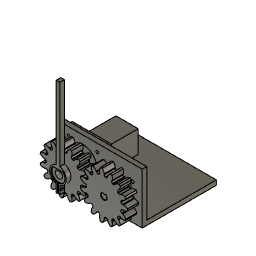
Encoder v10 (Autodesk Fusion 360 design; units mm, degrees)
description: Spur Gear; Module: 3.0; Num Teeth: 15; Pressure Angle: 20.0; Backlash: 0.00 mm
Autodesk Fusion 360 part; units mm, degrees
(part 1 of 6)
sketch "Sketch1" plane through (0, 0, 0) normal (0, 1, 0) x (1, 0, 0) in component "Motor"
  line L0 (0, 0) -> (-21.175, 0) construction
  line L1 (-21.175, 0) -> (-21.175, 21.175) construction
  line L2 (-21.175, 21.175) -> (0, 21.175) construction
  line L3 (0, 21.175) -> (0, 0) construction
  line L4 (-21.175, 21.175) -> (21.175, 21.175)
  line L5 (21.175, 21.175) -> (21.175, -21.175)
  line L6 (21.175, -21.175) -> (-21.175, -21.175)
  line L7 (-21.175, -21.175) -> (-21.175, 21.175)
  line L8 (0, 0) -> (-15.5, 0) construction
  line L9 (-15.5, 0) -> (-15.5, 15.5) construction
  line L10 (-15.5, 15.5) -> (0, 15.5) construction
  line L11 (0, 15.5) -> (0, 0) construction
  line L12 (-15.5, 15.5) -> (15.5, 15.5) construction
  line L13 (15.5, 15.5) -> (15.5, -15.5) construction
  line L14 (15.5, -15.5) -> (-15.5, -15.5) construction
  line L15 (-15.5, -15.5) -> (-15.5, 15.5) construction
  circle A0 centre (-15.5, 15.5) radius 1.5
  circle A1 centre (15.5, 15.5) radius 1.5
  circle A2 centre (-15.5, -15.5) radius 1.5
  circle A3 centre (15.5, -15.5) radius 1.5
  dimension "d68" = 21.175
  dimension "d69" = 21.175
  dimension "d70" = 42.35
  dimension "d71" = 42.35
  dimension "d72" = 15.5
  dimension "d73" = 15.5
  dimension "d74" = 31
  dimension "d75" = 31
  dimension "d76" = 3
  dimension "d77" = 3
  dimension "d78" = 3
  dimension "d79" = 3
  constraint horizontal L0
  constraint vertical L1
  constraint horizontal L2
  constraint vertical L3
  constraint coincident L0.start L3.end
  constraint horizontal L4
  constraint vertical L5
  constraint horizontal L6
  constraint vertical L7
  constraint horizontal L8
  constraint vertical L9
  constraint horizontal L10
  constraint vertical L11
  constraint horizontal L12
  constraint vertical L13
  constraint horizontal L14
  constraint vertical L15
  constraint coincident L9.end L10.start
  constraint coincident L12.end L13.start
  constraint coincident L14.end L15.start
  constraint coincident L13.end L14.start
  measures "d68" distance of L0.start L0.end
  measures "d69" distance of L0.start L2.end
  measures "d70" distance of L1.end L4.end
  measures "d71" distance of L1.end L6.end
  measures "d72" distance of L0.start L8.end
  measures "d73" distance of L0.start L10.end
  measures "d74" distance of L9.end L12.end
  measures "d75" distance of L9.end L14.end
  measures "d76" diameter of A0
  measures "d77" diameter of A1
  measures "d78" diameter of A2
  measures "d79" diameter of A3
extrude "Extrude1" add sketch "Sketch1" along normal blind 4.5 makes body 1 in component "Motor"
sketch "Sketch2" plane through (0, 4.5, 0) normal (0, 1, 0) x (-1, 0, 0) in component "Motor"
  circle A0 centre (15.5, -15.5) radius 1.5
  circle A1 centre (15.5, 15.5) radius 1.5
  circle A2 centre (-15.5, -15.5) radius 1.5
  circle A3 centre (-15.5, 15.5) radius 1.5
  line L0 (21.175, 21.175) -> (-21.175, 21.175)
  line L1 (-21.175, 21.175) -> (-21.175, -21.175)
  line L2 (-21.175, -21.175) -> (21.175, -21.175)
  line L3 (21.175, -21.175) -> (21.175, 21.175)
  line L4 (0, 0) -> (-12, 0) construction
  line L5 (-12, 0) -> (-12, -12) construction
  line L6 (-12, -12) -> (0, -12) construction
  line L7 (0, -12) -> (0, 0) construction
  line L8 (-12, -12) -> (12, -12)
  line L9 (12, -12) -> (12, 12)
  line L10 (12, 12) -> (-12, 12)
  line L11 (-12, 12) -> (-12, -12)
  dimension "d82" = 12
  dimension "d83" = 12
  dimension "d84" = 24
  dimension "d85" = 24
  constraint horizontal L4
  constraint vertical L5
  constraint horizontal L6
  constraint vertical L7
  constraint coincident L4.start L7.end
  constraint horizontal L8
  constraint vertical L9
  constraint horizontal L10
  constraint vertical L11
  measures "d82" distance of L4.start L4.end
  measures "d83" distance of L4.start L6.end
  measures "d84" distance of L5.end L8.end
  measures "d85" distance of L5.end L10.end
extrude "Extrude2" add sketch "Sketch2" along normal blind 38 contours L8 L9 L10 L11 bodies 1 in component "Motor"
sketch "Sketch3" plane through (0, 0, 0) normal (0, -1, 0) x (1, 0, 0) in component "Motor"
  circle A0 centre (-15.5, -15.5) radius 1.5
  circle A1 centre (-15.5, 15.5) radius 1.5
  circle A2 centre (15.5, -15.5) radius 1.5
  circle A3 centre (15.5, 15.5) radius 1.5
  line L0 (21.175, 21.175) -> (-21.175, 21.175)
  line L1 (-21.175, 21.175) -> (-21.175, -21.175)
  line L2 (-21.175, -21.175) -> (21.175, -21.175)
  line L3 (21.175, -21.175) -> (21.175, 21.175)
  circle A4 centre (0, 0) radius 12
  dimension "d88" = 24
  constraint coincident A4.centre origin
  measures "d88" diameter of A4
extrude "Extrude3" add sketch "Sketch3" along normal blind 2 contours A4 bodies 1 in component "Motor"
sketch "Sketch4" plane through (0, -2, 0) normal (0, -1, 0) x (1, 0, 0) in component "Motor"
  circle A0 centre (0, 0) radius 12
  circle A1 centre (0, 0) radius 4
  dimension "d91" = 8
  constraint coincident A0.centre A1.centre
  measures "d91" diameter of A1
extrude "Extrude4" add sketch "Sketch4" along normal blind 20 contours A1 bodies 1 in component "Motor"
sketch "Sketch1 (2)" plane through (0, 0, 0) normal (0, 1, 0) x (1, 0, 0) in component "encoder"
  line L0 (0, 0) -> (19, 0)
  line L1 (19, 0) -> (19, -26)
  line L2 (19, -26) -> (0, -26)
  line L3 (0, -26) -> (0, 0)
  line L4 (0, 0) -> (8, 0) construction
  line L5 (8, 0) -> (8, -12) construction
  line L6 (8, -12) -> (0, -12) construction
  line L7 (0, -12) -> (0, 0) construction
  line L8 (8, -12) -> (2.5, -12) construction
  line L9 (2.5, -12) -> (2.5, -6) construction
  line L10 (2.5, -6) -> (8, -6) construction
  line L11 (8, -6) -> (8, -12) construction
  line L12 (2.5, -6) -> (13.5, -6)
  line L13 (13.5, -6) -> (13.5, -18)
  line L14 (13.5, -18) -> (2.5, -18)
  line L15 (2.5, -18) -> (2.5, -6)
  dimension "d94" = 19
  dimension "d95" = 26
  dimension "d96" = 8
  dimension "d97" = 12
  dimension "d98" = 5.5
  dimension "d99" = 6
  dimension "d100" = 11
  dimension "d101" = 12
  constraint horizontal L0
  constraint vertical L1
  constraint horizontal L2
  constraint vertical L3
  constraint coincident L0.start L3.end
  constraint horizontal L4
  constraint vertical L5
  constraint horizontal L6
  constraint vertical L7
  constraint horizontal L8
  constraint vertical L9
  constraint horizontal L10
  constraint vertical L11
  constraint horizontal L12
  constraint vertical L13
  constraint horizontal L14
  constraint vertical L15
  measures "d94" distance of L0.start L0.end
  measures "d95" distance of L0.start L2.end
  measures "d96" distance of L0.start L4.end
  measures "d97" distance of L0.start L6.end
  measures "d98" distance of L5.end L8.end
  measures "d99" distance of L5.end L10.end
  measures "d100" distance of L9.end L12.end
  measures "d101" distance of L9.end L14.end
extrude "Extrude1'" add sketch "Sketch1 (2)" against normal blind 7 separate body contours L12 L13 L14 L15 makes body 2 in component "encoder"
extrude "Extrude2'" add sketch "Sketch1 (2)" along normal blind 1.2 separate body makes body 3 in component "encoder"
sketch "Sketch2 (2)" plane through (0, -7, 0) normal (0, -1, 0) x (1, 0, 0) in component "encoder"
  line L0 (13.5, 18) -> (2.5, 18)
  line L1 (2.5, 18) -> (2.5, 6)
  line L2 (2.5, 6) -> (13.5, 6)
  line L3 (13.5, 6) -> (13.5, 18)
  line L4 (2.5, 18) -> (13.5, 6) construction
  circle A0 centre (8, 12) radius 3
  dimension "d106" = 6
  constraint coincident L0.end L1.start
  constraint coincident L2.end L3.start
  constraint midpoint L4 A0.centre
  measures "d106" diameter of A0
extrude "Extrude3'" add sketch "Sketch2 (2)" along normal blind 20 contours A0 bodies 2 in component "encoder"
sketch "Sketch1 (3)" plane through (0, 0, 0) normal (0, 0, 1) x (1, 0, 0) in component "Spur Gear (15 teeth) (1)"
  circle A0 centre (0, 0) radius 18.8492
  circle A1 centre (0, 0) radius 4
extrude "Extrude1''" add sketch "Sketch1 (3)" along normal blind 12 separate body makes body 4 in component "Spur Gear (15 teeth) (1)"
sketch "Sketch2 (3)" plane through (0, 0, 0) normal (0, 0, 1) x (1, 0, 0) in component "Spur Gear (15 teeth) (1)"
  spline S0 degree 5 poles (20.992, -2.5232) (21.0048, -2.5247) (21.0305, -2.5274) (21.0691, -2.5303) (21.1207, -2.5321) (21.1854, -2.5313) (21.2502, -2.5284) (21.315, -2.5242) (21.38, -2.5193) (21.4449, -2.5139) (21.5099, -2.508) (21.575, -2.5014) (21.64, -2.4939) (21.7051, -2.4854) (21.7702, -2.4759) (21.8353, -2.4653) (21.9004, -2.454) (21.9656, -2.442) (22.0307, -2.4293) (22.0958, -2.4161) (22.1609, -2.4023) (22.226, -2.3879) (22.2911, -2.3729) (22.3562, -2.3572) (22.4212, -2.3409) (22.4862, -2.324) (22.5512, -2.3064) (22.6162, -2.2883) (22.6811, -2.2697) (22.746, -2.2505) (22.8109, -2.2308) (22.8757, -2.2106) (22.9405, -2.1898) (23.0053, -2.1685) (23.07, -2.1467) (23.1347, -2.1244) (23.1993, -2.1016) (23.2639, -2.0783) (23.3284, -2.0545) (23.3929, -2.0302) (23.4573, -2.0055) (23.5217, -1.9803) (23.586, -1.9546) (23.6502, -1.9284) (23.7144, -1.9018) (23.7785, -1.8747) (23.8426, -1.8472) (23.9066, -1.8192) (23.9705, -1.7908) (24.0344, -1.762) (24.0982, -1.7327) (24.1619, -1.703) (24.2255, -1.6729) (24.2891, -1.6423) (24.3526, -1.6113) (24.416, -1.5799) (24.4793, -1.5481) (24.5426, -1.5158) (24.6058, -1.4832) (24.6689, -1.4501) (24.7319, -1.4166) (24.7948, -1.3828) (24.8577, -1.3485) (24.9204, -1.3139) (24.9831, -1.2788) (25.0457, -1.2434) (25.1081, -1.2075) (25.1705, -1.1713) (25.2328, -1.1347) (25.295, -1.0977) (25.3571, -1.0603) (25.4067, -1.0301) (25.4439, -1.0073) (25.4686, -0.992) (25.481, -0.9843) knots 0 0 0 0 0 0 0.01428571 0.02857143 0.04285714 0.05714286 0.07142857 0.08571429 0.1 0.11428571 0.12857143 0.14285714 0.15714286 0.17142857 0.18571429 0.2 0.21428571 0.22857143 0.24285714 0.25714286 0.27142857 0.28571429 0.3 0.31428571 0.32857143 0.34285714 0.35714286 0.37142857 0.38571429 0.4 0.41428571 0.42857143 0.44285714 0.45714286 0.47142857 0.48571429 0.5 0.51428571 0.52857143 0.54285714 0.55714286 0.57142857 0.58571429 0.6 0.61428571 0.62857143 0.64285714 0.65714286 0.67142857 0.68571429 0.7 0.71428571 0.72857143 0.74285714 0.75714286 0.77142857 0.78571429 0.8 0.81428571 0.82857143 0.84285714 0.85714286 0.87142857 0.88571429 0.9 0.91428571 0.92857143 0.94285714 0.95714286 0.97142857 0.98571429 1 1 1 1 1 1
  spline S1 degree 5 poles (20.992, 2.5232) (21.0048, 2.5247) (21.0305, 2.5274) (21.0691, 2.5303) (21.1207, 2.5321) (21.1854, 2.5313) (21.2502, 2.5284) (21.315, 2.5242) (21.38, 2.5193) (21.4449, 2.5139) (21.5099, 2.508) (21.575, 2.5014) (21.64, 2.4939) (21.7051, 2.4854) (21.7702, 2.4759) (21.8353, 2.4653) (21.9004, 2.454) (21.9656, 2.442) (22.0307, 2.4293) (22.0958, 2.4161) (22.1609, 2.4023) (22.226, 2.3879) (22.2911, 2.3729) (22.3562, 2.3572) (22.4212, 2.3409) (22.4862, 2.324) (22.5512, 2.3064) (22.6162, 2.2883) (22.6811, 2.2697) (22.746, 2.2505) (22.8109, 2.2308) (22.8757, 2.2106) (22.9405, 2.1898) (23.0053, 2.1685) (23.07, 2.1467) (23.1347, 2.1244) (23.1993, 2.1016) (23.2639, 2.0783) (23.3284, 2.0545) (23.3929, 2.0302) (23.4573, 2.0055) (23.5217, 1.9803) (23.586, 1.9546) (23.6502, 1.9284) (23.7144, 1.9018) (23.7785, 1.8747) (23.8426, 1.8472) (23.9066, 1.8192) (23.9705, 1.7908) (24.0344, 1.762) (24.0982, 1.7327) (24.1619, 1.703) (24.2255, 1.6729) (24.2891, 1.6423) (24.3526, 1.6113) (24.416, 1.5799) (24.4793, 1.5481) (24.5426, 1.5158) (24.6058, 1.4832) (24.6689, 1.4501) (24.7319, 1.4166) (24.7948, 1.3828) (24.8577, 1.3485) (24.9204, 1.3139) (24.9831, 1.2788) (25.0457, 1.2434) (25.1081, 1.2075) (25.1705, 1.1713) (25.2328, 1.1347) (25.295, 1.0977) (25.3571, 1.0603) (25.4067, 1.0301) (25.4439, 1.0073) (25.4686, 0.992) (25.481, 0.9843) knots 0 0 0 0 0 0 0.01428571 0.02857143 0.04285714 0.05714286 0.07142857 0.08571429 0.1 0.11428571 0.12857143 0.14285714 0.15714286 0.17142857 0.18571429 0.2 0.21428571 0.22857143 0.24285714 0.25714286 0.27142857 0.28571429 0.3 0.31428571 0.32857143 0.34285714 0.35714286 0.37142857 0.38571429 0.4 0.41428571 0.42857143 0.44285714 0.45714286 0.47142857 0.48571429 0.5 0.51428571 0.52857143 0.54285714 0.55714286 0.57142857 0.58571429 0.6 0.61428571 0.62857143 0.64285714 0.65714286 0.67142857 0.68571429 0.7 0.71428571 0.72857143 0.74285714 0.75714286 0.77142857 0.78571429 0.8 0.81428571 0.82857143 0.84285714 0.85714286 0.87142857 0.88571429 0.9 0.91428571 0.92857143 0.94285714 0.95714286 0.97142857 0.98571429 1 1 1 1 1 1
  arc A0 (25.481, -0.9843) -> (25.481, 0.9843) centre (0, 0) ccw
  line L0 (18.7046, -2.2494) -> (20.992, -2.5232)
  line L1 (18.7046, 2.2494) -> (20.992, 2.5232)
  line L2 (18.7046, -2.2494) -> (18.7046, 2.2494)
  point P0 (21.3052, -2.5247)
  point P1 (21.6219, -2.4959)
  point P2 (21.9407, -2.4465)
  point P3 (22.2611, -2.3798)
  point P4 (22.5825, -2.2976)
  point P5 (22.9048, -2.2012)
  point P6 (23.2276, -2.0913)
  point P7 (23.5506, -1.9686)
  point P8 (23.8736, -1.8336)
  point P9 (24.1965, -1.6866)
  point P10 (24.5188, -1.5279)
  point P11 (24.8405, -1.3578)
  point P12 (25.1613, -1.1766)
  point P13 (21.3052, 2.5247)
  point P14 (21.6219, 2.4959)
  point P15 (21.9407, 2.4465)
  point P16 (22.2611, 2.3798)
  point P17 (22.5825, 2.2976)
  point P18 (22.9048, 2.2012)
  point P19 (23.2276, 2.0913)
  point P20 (23.5506, 1.9686)
  point P21 (23.8736, 1.8336)
  point P22 (24.1965, 1.6866)
  point P23 (24.5188, 1.5279)
  point P24 (24.8405, 1.3578)
  point P25 (25.1613, 1.1766)
extrude "Extrude2''" add sketch "Sketch2 (3)" along normal blind 12 bodies 4 in component "Spur Gear (15 teeth) (1)"
fillet "Fillet1" radius 1.5 2 edges at (18.7144, -2.2506, 6) (18.7144, 2.2506, 6) on bodies 4 in component "Spur Gear (15 teeth) (1)"
pattern_circular "C-Pattern1" count 15 over 360 about axis through (0, 0, 0) along (0, 0, 1) of "Extrude2''", "Fillet1" in component "Spur Gear (15 teeth) (1)"
sketch "Sketch3 (2)" plane through (0, 0, 0) normal (0, 0, 1) x (1, 0, 0) in component "Spur Gear (15 teeth) (1)"
  circle A0 centre (0, 0) radius 22.5 construction
sketch "Sketch1 (4)" plane through (0, 0, 0) normal (0, 0, 1) x (1, 0, 0) in component "Spur Gear (15 teeth)"
  circle A0 centre (0, 0) radius 18.8492
  circle A1 centre (0, 0) radius 3.5
  dimension "d237" = 7
  measures "d237" diameter of A1
extrude "Extrude1'''" add sketch "Sketch1 (4)" along normal blind 12 separate body makes body 5 in component "Spur Gear (15 teeth)"
sketch "Sketch2 (4)" plane through (0, 0, 0) normal (0, 0, 1) x (1, 0, 0) in component "Spur Gear (15 teeth)"
  spline S0 degree 5 poles (20.992, -2.5232) (21.0048, -2.5247) (21.0305, -2.5274) (21.0691, -2.5303) (21.1207, -2.5321) (21.1854, -2.5313) (21.2502, -2.5284) (21.315, -2.5242) (21.38, -2.5193) (21.4449, -2.5139) (21.5099, -2.508) (21.575, -2.5014) (21.64, -2.4939) (21.7051, -2.4854) (21.7702, -2.4759) (21.8353, -2.4653) (21.9004, -2.454) (21.9656, -2.442) (22.0307, -2.4293) (22.0958, -2.4161) (22.1609, -2.4023) (22.226, -2.3879) (22.2911, -2.3729) (22.3562, -2.3572) (22.4212, -2.3409) (22.4862, -2.324) (22.5512, -2.3064) (22.6162, -2.2883) (22.6811, -2.2697) (22.746, -2.2505) (22.8109, -2.2308) (22.8757, -2.2106) (22.9405, -2.1898) (23.0053, -2.1685) (23.07, -2.1467) (23.1347, -2.1244) (23.1993, -2.1016) (23.2639, -2.0783) (23.3284, -2.0545) (23.3929, -2.0302) (23.4573, -2.0055) (23.5217, -1.9803) (23.586, -1.9546) (23.6502, -1.9284) (23.7144, -1.9018) (23.7785, -1.8747) (23.8426, -1.8472) (23.9066, -1.8192) (23.9705, -1.7908) (24.0344, -1.762) (24.0982, -1.7327) (24.1619, -1.703) (24.2255, -1.6729) (24.2891, -1.6423) (24.3526, -1.6113) (24.416, -1.5799) (24.4793, -1.5481) (24.5426, -1.5158) (24.6058, -1.4832) (24.6689, -1.4501) (24.7319, -1.4166) (24.7948, -1.3828) (24.8577, -1.3485) (24.9204, -1.3139) (24.9831, -1.2788) (25.0457, -1.2434) (25.1081, -1.2075) (25.1705, -1.1713) (25.2328, -1.1347) (25.295, -1.0977) (25.3571, -1.0603) (25.4067, -1.0301) (25.4439, -1.0073) (25.4686, -0.992) (25.481, -0.9843) knots 0 0 0 0 0 0 0.01428571 0.02857143 0.04285714 0.05714286 0.07142857 0.08571429 0.1 0.11428571 0.12857143 0.14285714 0.15714286 0.17142857 0.18571429 0.2 0.21428571 0.22857143 0.24285714 0.25714286 0.27142857 0.28571429 0.3 0.31428571 0.32857143 0.34285714 0.35714286 0.37142857 0.38571429 0.4 0.41428571 0.42857143 0.44285714 0.45714286 0.47142857 0.48571429 0.5 0.51428571 0.52857143 0.54285714 0.55714286 0.57142857 0.58571429 0.6 0.61428571 0.62857143 0.64285714 0.65714286 0.67142857 0.68571429 0.7 0.71428571 0.72857143 0.74285714 0.75714286 0.77142857 0.78571429 0.8 0.81428571 0.82857143 0.84285714 0.85714286 0.87142857 0.88571429 0.9 0.91428571 0.92857143 0.94285714 0.95714286 0.97142857 0.98571429 1 1 1 1 1 1
  spline S1 degree 5 poles (20.992, 2.5232) (21.0048, 2.5247) (21.0305, 2.5274) (21.0691, 2.5303) (21.1207, 2.5321) (21.1854, 2.5313) (21.2502, 2.5284) (21.315, 2.5242) (21.38, 2.5193) (21.4449, 2.5139) (21.5099, 2.508) (21.575, 2.5014) (21.64, 2.4939) (21.7051, 2.4854) (21.7702, 2.4759) (21.8353, 2.4653) (21.9004, 2.454) (21.9656, 2.442) (22.0307, 2.4293) (22.0958, 2.4161) (22.1609, 2.4023) (22.226, 2.3879) (22.2911, 2.3729) (22.3562, 2.3572) (22.4212, 2.3409) (22.4862, 2.324) (22.5512, 2.3064) (22.6162, 2.2883) (22.6811, 2.2697) (22.746, 2.2505) (22.8109, 2.2308) (22.8757, 2.2106) (22.9405, 2.1898) (23.0053, 2.1685) (23.07, 2.1467) (23.1347, 2.1244) (23.1993, 2.1016) (23.2639, 2.0783) (23.3284, 2.0545) (23.3929, 2.0302) (23.4573, 2.0055) (23.5217, 1.9803) (23.586, 1.9546) (23.6502, 1.9284) (23.7144, 1.9018) (23.7785, 1.8747) (23.8426, 1.8472) (23.9066, 1.8192) (23.9705, 1.7908) (24.0344, 1.762) (24.0982, 1.7327) (24.1619, 1.703) (24.2255, 1.6729) (24.2891, 1.6423) (24.3526, 1.6113) (24.416, 1.5799) (24.4793, 1.5481) (24.5426, 1.5158) (24.6058, 1.4832) (24.6689, 1.4501) (24.7319, 1.4166) (24.7948, 1.3828) (24.8577, 1.3485) (24.9204, 1.3139) (24.9831, 1.2788) (25.0457, 1.2434) (25.1081, 1.2075) (25.1705, 1.1713) (25.2328, 1.1347) (25.295, 1.0977) (25.3571, 1.0603) (25.4067, 1.0301) (25.4439, 1.0073) (25.4686, 0.992) (25.481, 0.9843) knots 0 0 0 0 0 0 0.01428571 0.02857143 0.04285714 0.05714286 0.07142857 0.08571429 0.1 0.11428571 0.12857143 0.14285714 0.15714286 0.17142857 0.18571429 0.2 0.21428571 0.22857143 0.24285714 0.25714286 0.27142857 0.28571429 0.3 0.31428571 0.32857143 0.34285714 0.35714286 0.37142857 0.38571429 0.4 0.41428571 0.42857143 0.44285714 0.45714286 0.47142857 0.48571429 0.5 0.51428571 0.52857143 0.54285714 0.55714286 0.57142857 0.58571429 0.6 0.61428571 0.62857143 0.64285714 0.65714286 0.67142857 0.68571429 0.7 0.71428571 0.72857143 0.74285714 0.75714286 0.77142857 0.78571429 0.8 0.81428571 0.82857143 0.84285714 0.85714286 0.87142857 0.88571429 0.9 0.91428571 0.92857143 0.94285714 0.95714286 0.97142857 0.98571429 1 1 1 1 1 1
  arc A0 (25.481, -0.9843) -> (25.481, 0.9843) centre (0, 0) ccw
  line L0 (18.7046, -2.2494) -> (20.992, -2.5232)
  line L1 (18.7046, 2.2494) -> (20.992, 2.5232)
  line L2 (18.7046, -2.2494) -> (18.7046, 2.2494)
  point P0 (21.3052, -2.5247)
  point P1 (21.6219, -2.4959)
  point P2 (21.9407, -2.4465)
  point P3 (22.2611, -2.3798)
  point P4 (22.5825, -2.2976)
  point P5 (22.9048, -2.2012)
  point P6 (23.2276, -2.0913)
  point P7 (23.5506, -1.9686)
  point P8 (23.8736, -1.8336)
  point P9 (24.1965, -1.6866)
  point P10 (24.5188, -1.5279)
  point P11 (24.8405, -1.3578)
  point P12 (25.1613, -1.1766)
  point P13 (21.3052, 2.5247)
  point P14 (21.6219, 2.4959)
  point P15 (21.9407, 2.4465)
  point P16 (22.2611, 2.3798)
  point P17 (22.5825, 2.2976)
  point P18 (22.9048, 2.2012)
  point P19 (23.2276, 2.0913)
  point P20 (23.5506, 1.9686)
  point P21 (23.8736, 1.8336)
  point P22 (24.1965, 1.6866)
  point P23 (24.5188, 1.5279)
  point P24 (24.8405, 1.3578)
  point P25 (25.1613, 1.1766)
extrude "Extrude2'''" add sketch "Sketch2 (4)" along normal blind 12 bodies 5 in component "Spur Gear (15 teeth)"
fillet "Fillet1'" radius 1.5 2 edges at (18.7144, -2.2506, 6) (18.7144, 2.2506, 6) on bodies 5 in component "Spur Gear (15 teeth)"
pattern_circular "C-Pattern1'" count 15 over 360 about axis through (0, 0, 0) along (0, 0, 1) of "Extrude2'''", "Fillet1'" in component "Spur Gear (15 teeth)"
sketch "Sketch3 (3)" plane through (0, 0, 0) normal (0, 0, 1) x (1, 0, 0) in component "Spur Gear (15 teeth)"
  circle A0 centre (0, 0) radius 22.5 construction
sketch "Sketch1 (5)" plane through (0, 0, 0) normal (0, -1, 0) x (1, 0, 0) in component "Body"
  circle A0 centre (0, 0) radius 12
  circle A1 centre (-15.5, -15.5) radius 1.5
  circle A2 centre (-15.5, 15.5) radius 1.5
  circle A3 centre (15.5, -15.5) radius 1.5
  circle A4 centre (15.5, 15.5) radius 1.5
  line L0 (21.175, 21.175) -> (-21.175, 21.175)
  line L1 (-21.175, 21.175) -> (-21.175, -21.175)
  line L2 (-21.175, -21.175) -> (21.175, -21.175)
  line L3 (21.175, -21.175) -> (21.175, 21.175)
  line L4 (-21.175, -21.175) -> (-26.175, -21.175) construction
  line L5 (-26.175, -21.175) -> (-26.175, -26.175) construction
  line L6 (-26.175, -26.175) -> (-21.175, -26.175) construction
  line L7 (-21.175, -26.175) -> (-21.175, -21.175) construction
  line L8 (-26.175, -26.175) -> (63.825, -26.175)
  line L9 (63.825, -26.175) -> (63.825, 23.825)
  line L10 (63.825, 23.825) -> (-26.175, 23.825)
  line L11 (-26.175, 23.825) -> (-26.175, -26.175)
  dimension "d141" = 5
  dimension "d142" = 5
  dimension "d143" = 90
  dimension "d144" = 50
  constraint horizontal L4
  constraint vertical L5
  constraint horizontal L6
  constraint vertical L7
  constraint coincident L1.end L2.start
  constraint horizontal L8
  constraint vertical L9
  constraint horizontal L10
  constraint vertical L11
  measures "d141" distance of L1.end L4.end
  measures "d142" distance of L1.end L6.end
  measures "d143" distance of L5.end L8.end
  measures "d144" distance of L5.end L10.end
extrude "Extrude1''''" add sketch "Sketch1 (5)" against normal blind 5 separate body contours A0 | L0 L1 L2 L3 | L8 L9 L10 L11 makes body 6 in component "Body"
sketch "Sketch2 (5)" plane through (0, -11, 0) normal (0, -1, 0) x (1, 0, 0) in component "Body"
  circle A0 centre (0, 0) radius 4
  circle A1 centre (0, 0) radius 15
  dimension "d147" = 30
  constraint coincident A0.centre A1.centre
  measures "d147" diameter of A1
extrude "Extrude2''''" cut sketch "Sketch2 (5)" against normal blind 16 contours A0 | A1 bodies 6 in component "Body"
sketch "Sketch3 (4)" plane through (0, 8.3, 0) normal (0, 1, 0) x (-1, 0, 0) in component "Body"
  line L0 (-39.2194, 6) -> (-50.2194, 6)
  line L1 (-50.2194, 6) -> (-50.2194, -6)
  line L2 (-50.2194, -6) -> (-39.2194, -6)
  line L3 (-39.2194, -6) -> (-39.2194, 6)
  line L4 (-51.7194, -7.5) -> (-37.7194, -7.5)
  line L5 (-37.7194, -7.5) -> (-37.7194, 7.5)
  line L6 (-37.7194, 7.5) -> (-51.7194, 7.5)
  line L7 (-51.7194, 7.5) -> (-51.7194, -7.5)
  dimension "d150" = 1.5
extrude "Extrude3''" cut sketch "Sketch3 (4)" against normal blind 8.3 contours L0 L1 L2 L3 | L4 L5 L6 L7 bodies 6 in component "Body"
extrude "Extrude4'" add 1 faces at (6.1667, 0, 10) along direction (0, 1, 0) blind 1.2 on bodies 2 bodies 2 3 in component "encoder"
sketch "Sketch4 (2)" plane through (0, 0, 0) normal (0, -1, 0) x (1, 0, 0) in component "Body"
  line L0 (51.7194, -7.5) -> (37.7194, -7.5)
  line L1 (37.7194, -7.5) -> (37.7194, 7.5)
  line L2 (37.7194, 7.5) -> (51.7194, 7.5)
  line L3 (51.7194, 7.5) -> (51.7194, -7.5)
  circle A0 centre (0, 0) radius 15
  circle A1 centre (15.5, 15.5) radius 1.5
  circle A2 centre (-15.5, -15.5) radius 1.5
  circle A3 centre (15.5, -15.5) radius 1.5
  circle A4 centre (-15.5, 15.5) radius 1.5
  line L4 (-26.175, 23.825) -> (-26.175, -26.175)
  line L5 (-26.175, -26.175) -> (63.825, -26.175)
  line L6 (63.825, -26.175) -> (63.825, 23.825)
  line L7 (63.825, 23.825) -> (-26.175, 23.825)
  line L8 (-26.175, -26.175) -> (63.825, -26.175)
  line L9 (63.825, -26.175) -> (63.825, -31.175)
  line L10 (63.825, -31.175) -> (-26.175, -31.175)
  line L11 (-26.175, -31.175) -> (-26.175, -26.175)
  dimension "d197" = 90
  dimension "d198" = 5
  constraint horizontal L8
  constraint vertical L9
  constraint horizontal L10
  constraint vertical L11
  constraint coincident L4.end L5.start
  measures "d197" distance of L4.end L5.end
  measures "d198" distance of L4.end L10.end
sketch "Sketch4 (3)" plane through (0, 0, 12) normal (0, 0, 1) x (-1, 0, 0) in component "Spur Gear (15 teeth) (1)"
  arc A0 (-18.3722, 4.2137) -> (-18.4977, 3.6232) centre (0, 0) ccw
  arc A1 (-20.148, 2.4222) -> (-18.4977, 3.6232) centre (-19.9697, 3.9116) ccw
  line L0 (-20.148, 2.4222) -> (-20.992, 2.5232)
  spline S0 degree 5 poles (-20.992, 2.5232) (-21.0048, 2.5247) (-21.0305, 2.5274) (-21.0691, 2.5303) (-21.1207, 2.5321) (-21.1854, 2.5313) (-21.2502, 2.5284) (-21.315, 2.5242) (-21.38, 2.5193) (-21.4449, 2.5139) (-21.5099, 2.508) (-21.575, 2.5014) (-21.64, 2.4939) (-21.7051, 2.4854) (-21.7702, 2.4759) (-21.8353, 2.4653) (-21.9004, 2.454) (-21.9656, 2.442) (-22.0307, 2.4293) (-22.0958, 2.4161) (-22.1609, 2.4023) (-22.226, 2.3879) (-22.2911, 2.3729) (-22.3562, 2.3572) (-22.4212, 2.3409) (-22.4862, 2.324) (-22.5512, 2.3064) (-22.6162, 2.2883) (-22.6811, 2.2697) (-22.746, 2.2505) (-22.8109, 2.2308) (-22.8757, 2.2106) (-22.9405, 2.1898) (-23.0053, 2.1685) (-23.07, 2.1467) (-23.1347, 2.1244) (-23.1993, 2.1016) (-23.2639, 2.0783) (-23.3284, 2.0545) (-23.3929, 2.0302) (-23.4573, 2.0055) (-23.5217, 1.9803) (-23.586, 1.9546) (-23.6502, 1.9284) (-23.7144, 1.9018) (-23.7785, 1.8747) (-23.8426, 1.8472) (-23.9066, 1.8192) (-23.9705, 1.7908) (-24.0344, 1.762) (-24.0982, 1.7327) (-24.1619, 1.703) (-24.2255, 1.6729) (-24.2891, 1.6423) (-24.3526, 1.6113) (-24.416, 1.5799) (-24.4793, 1.5481) (-24.5426, 1.5158) (-24.6058, 1.4832) (-24.6689, 1.4501) (-24.7319, 1.4166) (-24.7948, 1.3828) (-24.8577, 1.3485) (-24.9204, 1.3139) (-24.9831, 1.2788) (-25.0457, 1.2434) (-25.1081, 1.2075) (-25.1705, 1.1713) (-25.2328, 1.1347) (-25.295, 1.0977) (-25.3571, 1.0603) (-25.4067, 1.0301) (-25.4439, 1.0073) (-25.4686, 0.992) (-25.481, 0.9843) knots 0 0 0 0 0 0 0.01428571 0.02857143 0.04285714 0.05714286 0.07142857 0.08571429 0.1 0.11428571 0.12857143 0.14285714 0.15714286 0.17142857 0.18571429 0.2 0.21428571 0.22857143 0.24285714 0.25714286 0.27142857 0.28571429 0.3 0.31428571 0.32857143 0.34285714 0.35714286 0.37142857 0.38571429 0.4 0.41428571 0.42857143 0.44285714 0.45714286 0.47142857 0.48571429 0.5 0.51428571 0.52857143 0.54285714 0.55714286 0.57142857 0.58571429 0.6 0.61428571 0.62857143 0.64285714 0.65714286 0.67142857 0.68571429 0.7 0.71428571 0.72857143 0.74285714 0.75714286 0.77142857 0.78571429 0.8 0.81428571 0.82857143 0.84285714 0.85714286 0.87142857 0.88571429 0.9 0.91428571 0.92857143 0.94285714 0.95714286 0.97142857 0.98571429 1 1 1 1 1 1
  arc A2 (-25.481, 0.9843) -> (-25.481, -0.9843) centre (0, 0) ccw
  spline S1 degree 5 poles (-25.481, -0.9843) (-25.4686, -0.992) (-25.4439, -1.0073) (-25.4067, -1.0301) (-25.3571, -1.0603) (-25.295, -1.0977) (-25.2328, -1.1347) (-25.1705, -1.1713) (-25.1081, -1.2075) (-25.0457, -1.2434) (-24.9831, -1.2788) (-24.9204, -1.3139) (-24.8577, -1.3485) (-24.7948, -1.3828) (-24.7319, -1.4166) (-24.6689, -1.4501) (-24.6058, -1.4832) (-24.5426, -1.5158) (-24.4793, -1.5481) (-24.416, -1.5799) (-24.3526, -1.6113) (-24.2891, -1.6423) (-24.2255, -1.6729) (-24.1619, -1.703) (-24.0982, -1.7327) (-24.0344, -1.762) (-23.9705, -1.7908) (-23.9066, -1.8192) (-23.8426, -1.8472) (-23.7785, -1.8747) (-23.7144, -1.9018) (-23.6502, -1.9284) (-23.586, -1.9546) (-23.5217, -1.9803) (-23.4573, -2.0055) (-23.3929, -2.0302) (-23.3284, -2.0545) (-23.2639, -2.0783) (-23.1993, -2.1016) (-23.1347, -2.1244) (-23.07, -2.1467) (-23.0053, -2.1685) (-22.9405, -2.1898) (-22.8757, -2.2106) (-22.8109, -2.2308) (-22.746, -2.2505) (-22.6811, -2.2697) (-22.6162, -2.2883) (-22.5512, -2.3064) (-22.4862, -2.324) (-22.4212, -2.3409) (-22.3562, -2.3572) (-22.2911, -2.3729) (-22.226, -2.3879) (-22.1609, -2.4023) (-22.0958, -2.4161) (-22.0307, -2.4293) (-21.9656, -2.442) (-21.9004, -2.454) (-21.8353, -2.4653) (-21.7702, -2.4759) (-21.7051, -2.4854) (-21.64, -2.4939) (-21.575, -2.5014) (-21.5099, -2.508) (-21.4449, -2.5139) (-21.38, -2.5193) (-21.315, -2.5242) (-21.2502, -2.5284) (-21.1854, -2.5313) (-21.1207, -2.5321) (-21.0691, -2.5303) (-21.0305, -2.5274) (-21.0048, -2.5247) (-20.992, -2.5232) knots -1 -1 -1 -1 -1 -1 -0.98571429 -0.97142857 -0.95714286 -0.94285714 -0.92857143 -0.91428571 -0.9 -0.88571429 -0.87142857 -0.85714286 -0.84285714 -0.82857143 -0.81428571 -0.8 -0.78571429 -0.77142857 -0.75714286 -0.74285714 -0.72857143 -0.71428571 -0.7 -0.68571429 -0.67142857 -0.65714286 -0.64285714 -0.62857143 -0.61428571 -0.6 -0.58571429 -0.57142857 -0.55714286 -0.54285714 -0.52857143 -0.51428571 -0.5 -0.48571429 -0.47142857 -0.45714286 -0.44285714 -0.42857143 -0.41428571 -0.4 -0.38571429 -0.37142857 -0.35714286 -0.34285714 -0.32857143 -0.31428571 -0.3 -0.28571429 -0.27142857 -0.25714286 -0.24285714 -0.22857143 -0.21428571 -0.2 -0.18571429 -0.17142857 -0.15714286 -0.14285714 -0.12857143 -0.11428571 -0.1 -0.08571429 -0.07142857 -0.05714286 -0.04285714 -0.02857143 -0.01428571 0 0 0 0 0 0
  line L1 (-20.992, -2.5232) -> (-20.148, -2.4222)
  arc A3 (-18.4977, -3.6232) -> (-20.148, -2.4222) centre (-19.9697, -3.9116) ccw
  arc A4 (-18.4977, -3.6232) -> (-18.3722, -4.2137) centre (0, 0) ccw
  arc A5 (-19.3913, -5.9821) -> (-18.3722, -4.2137) centre (-19.8342, -4.549) ccw
  line L2 (-19.3913, -5.9821) -> (-20.2034, -6.2332)
  spline S2 degree 5 poles (-20.2034, -6.2332) (-20.2158, -6.237) (-20.2403, -6.245) (-20.2768, -6.258) (-20.3246, -6.2774) (-20.3834, -6.3044) (-20.4414, -6.3334) (-20.4989, -6.3636) (-20.5563, -6.3945) (-20.6134, -6.4259) (-20.6704, -6.4577) (-20.7271, -6.4902) (-20.7835, -6.5235) (-20.8395, -6.5577) (-20.8951, -6.5929) (-20.9503, -6.629) (-21.0052, -6.6659) (-21.0598, -6.7034) (-21.1141, -6.7414) (-21.1683, -6.7799) (-21.2221, -6.819) (-21.2757, -6.8586) (-21.3291, -6.8988) (-21.3821, -6.9396) (-21.4349, -6.981) (-21.4874, -7.0229) (-21.5397, -7.0654) (-21.5917, -7.1084) (-21.6434, -7.1518) (-21.6949, -7.1957) (-21.7462, -7.2401) (-21.7972, -7.2849) (-21.8479, -7.3303) (-21.8984, -7.376) (-21.9487, -7.4223) (-21.9987, -7.469) (-22.0484, -7.5161) (-22.0979, -7.5637) (-22.1472, -7.6116) (-22.1962, -7.66) (-22.245, -7.7088) (-22.2935, -7.7581) (-22.3418, -7.8077) (-22.3899, -7.8577) (-22.4377, -7.9081) (-22.4853, -7.9589) (-22.5326, -8.0101) (-22.5797, -8.0617) (-22.6265, -8.1137) (-22.6731, -8.166) (-22.7195, -8.2187) (-22.7656, -8.2718) (-22.8115, -8.3252) (-22.8572, -8.379) (-22.9026, -8.4331) (-22.9477, -8.4876) (-22.9926, -8.5424) (-23.0373, -8.5976) (-23.0818, -8.6531) (-23.126, -8.709) (-23.1699, -8.7652) (-23.2136, -8.8217) (-23.2571, -8.8786) (-23.3003, -8.9358) (-23.3433, -8.9933) (-23.3861, -9.0511) (-23.4286, -9.1093) (-23.4708, -9.1677) (-23.5128, -9.2265) (-23.5546, -9.2856) (-23.5961, -9.345) (-23.6292, -9.3928) (-23.6538, -9.4287) (-23.6702, -9.4528) (-23.6784, -9.4648) knots 0 0 0 0 0 0 0.01428571 0.02857143 0.04285714 0.05714286 0.07142857 0.08571429 0.1 0.11428571 0.12857143 0.14285714 0.15714286 0.17142857 0.18571429 0.2 0.21428571 0.22857143 0.24285714 0.25714286 0.27142857 0.28571429 0.3 0.31428571 0.32857143 0.34285714 0.35714286 0.37142857 0.38571429 0.4 0.41428571 0.42857143 0.44285714 0.45714286 0.47142857 0.48571429 0.5 0.51428571 0.52857143 0.54285714 0.55714286 0.57142857 0.58571429 0.6 0.61428571 0.62857143 0.64285714 0.65714286 0.67142857 0.68571429 0.7 0.71428571 0.72857143 0.74285714 0.75714286 0.77142857 0.78571429 0.8 0.81428571 0.82857143 0.84285714 0.85714286 0.87142857 0.88571429 0.9 0.91428571 0.92857143 0.94285714 0.95714286 0.97142857 0.98571429 1 1 1 1 1 1
  arc A6 (-23.6784, -9.4648) -> (-22.8777, -11.2633) centre (0, 0) ccw
  spline S3 degree 5 poles (-22.8777, -11.2633) (-22.8633, -11.2653) (-22.8344, -11.2692) (-22.7912, -11.2749) (-22.7336, -11.2823) (-22.6617, -11.2912) (-22.5898, -11.2997) (-22.518, -11.3078) (-22.4463, -11.3155) (-22.3746, -11.3228) (-22.303, -11.3298) (-22.2315, -11.3363) (-22.1601, -11.3425) (-22.0888, -11.3482) (-22.0175, -11.3535) (-21.9463, -11.3585) (-21.8752, -11.363) (-21.8043, -11.3671) (-21.7333, -11.3709) (-21.6625, -11.3742) (-21.5918, -11.3771) (-21.5212, -11.3796) (-21.4507, -11.3816) (-21.3803, -11.3833) (-21.31, -11.3845) (-21.2398, -11.3853) (-21.1697, -11.3857) (-21.0998, -11.3856) (-21.0299, -11.3852) (-20.9602, -11.3842) (-20.8906, -11.3829) (-20.8212, -11.3811) (-20.7518, -11.3789) (-20.6827, -11.3762) (-20.6136, -11.373) (-20.5447, -11.3694) (-20.4759, -11.3654) (-20.4073, -11.3609) (-20.3388, -11.3559) (-20.2705, -11.3505) (-20.2023, -11.3446) (-20.1344, -11.3381) (-20.0665, -11.3313) (-19.9989, -11.3239) (-19.9315, -11.316) (-19.8642, -11.3076) (-19.7971, -11.2987) (-19.7302, -11.2893) (-19.6635, -11.2794) (-19.597, -11.269) (-19.5307, -11.258) (-19.4646, -11.2465) (-19.3988, -11.2344) (-19.3332, -11.2216) (-19.2679, -11.2083) (-19.2028, -11.1944) (-19.138, -11.18) (-19.0733, -11.165) (-19.0089, -11.1495) (-18.9448, -11.1334) (-18.881, -11.1165) (-18.8177, -11.0988) (-18.7548, -11.0801) (-18.6923, -11.0605) (-18.6302, -11.0401) (-18.5684, -11.019) (-18.5069, -10.9975) (-18.4456, -10.9756) (-18.3846, -10.953) (-18.3242, -10.9293) (-18.2648, -10.9037) (-18.2184, -10.8812) (-18.1843, -10.8628) (-18.162, -10.8499) (-18.1509, -10.8433) knots -1 -1 -1 -1 -1 -1 -0.98571429 -0.97142857 -0.95714286 -0.94285714 -0.92857143 -0.91428571 -0.9 -0.88571429 -0.87142857 -0.85714286 -0.84285714 -0.82857143 -0.81428571 -0.8 -0.78571429 -0.77142857 -0.75714286 -0.74285714 -0.72857143 -0.71428571 -0.7 -0.68571429 -0.67142857 -0.65714286 -0.64285714 -0.62857143 -0.61428571 -0.6 -0.58571429 -0.57142857 -0.55714286 -0.54285714 -0.52857143 -0.51428571 -0.5 -0.48571429 -0.47142857 -0.45714286 -0.44285714 -0.42857143 -0.41428571 -0.4 -0.38571429 -0.37142857 -0.35714286 -0.34285714 -0.32857143 -0.31428571 -0.3 -0.28571429 -0.27142857 -0.25714286 -0.24285714 -0.22857143 -0.21428571 -0.2 -0.18571429 -0.17142857 -0.15714286 -0.14285714 -0.12857143 -0.11428571 -0.1 -0.08571429 -0.07142857 -0.05714286 -0.04285714 -0.02857143 -0.01428571 0 0 0 0 0 0
  line L3 (-18.1509, -10.8433) -> (-17.4209, -10.4077)
  arc A7 (-15.4248, -10.8337) -> (-17.4209, -10.4077) centre (-16.6523, -11.6958) ccw
  arc A8 (-15.4248, -10.8337) -> (-15.07, -11.3221) centre (0, 0) ccw
  arc A9 (-15.2817, -13.3521) -> (-15.07, -11.3221) centre (-16.2692, -12.223) ccw
  line L4 (-15.2817, -13.3521) -> (-15.9215, -13.9117)
  spline S4 degree 5 poles (-15.9215, -13.9117) (-15.9312, -13.9202) (-15.9504, -13.9375) (-15.9784, -13.9643) (-16.0142, -14.0015) (-16.0569, -14.05) (-16.0981, -14.1001) (-16.1384, -14.1511) (-16.1782, -14.2027) (-16.2177, -14.2546) (-16.2568, -14.3068) (-16.2954, -14.3595) (-16.3334, -14.4129) (-16.3706, -14.467) (-16.407, -14.5217) (-16.4428, -14.5772) (-16.4779, -14.6332) (-16.5126, -14.6896) (-16.5468, -14.7465) (-16.5805, -14.8037) (-16.6138, -14.8613) (-16.6467, -14.9193) (-16.6791, -14.9777) (-16.711, -15.0366) (-16.7423, -15.0958) (-16.7733, -15.1555) (-16.8037, -15.2155) (-16.8337, -15.2759) (-16.8633, -15.3367) (-16.8925, -15.3977) (-16.9213, -15.4591) (-16.9496, -15.5208) (-16.9776, -15.5829) (-17.0051, -15.6452) (-17.0322, -15.7079) (-17.0589, -15.7709) (-17.0852, -15.8342) (-17.111, -15.8978) (-17.1365, -15.9617) (-17.1616, -16.0258) (-17.1863, -16.0902) (-17.2107, -16.1549) (-17.2346, -16.2199) (-17.2582, -16.2852) (-17.2813, -16.3507) (-17.3041, -16.4164) (-17.3265, -16.4825) (-17.3486, -16.5487) (-17.3702, -16.6152) (-17.3915, -16.682) (-17.4125, -16.749) (-17.433, -16.8162) (-17.4532, -16.8837) (-17.473, -16.9514) (-17.4925, -17.0193) (-17.5116, -17.0875) (-17.5303, -17.1558) (-17.5487, -17.2244) (-17.5667, -17.2932) (-17.5843, -17.3622) (-17.6016, -17.4315) (-17.6186, -17.5009) (-17.6352, -17.5705) (-17.6514, -17.6403) (-17.6673, -17.7104) (-17.6828, -17.7806) (-17.698, -17.851) (-17.7128, -17.9216) (-17.7273, -17.9924) (-17.7414, -18.0634) (-17.7552, -18.1345) (-17.7659, -18.1916) (-17.7738, -18.2345) (-17.779, -18.2631) (-17.7816, -18.2774) knots 0 0 0 0 0 0 0.01428571 0.02857143 0.04285714 0.05714286 0.07142857 0.08571429 0.1 0.11428571 0.12857143 0.14285714 0.15714286 0.17142857 0.18571429 0.2 0.21428571 0.22857143 0.24285714 0.25714286 0.27142857 0.28571429 0.3 0.31428571 0.32857143 0.34285714 0.35714286 0.37142857 0.38571429 0.4 0.41428571 0.42857143 0.44285714 0.45714286 0.47142857 0.48571429 0.5 0.51428571 0.52857143 0.54285714 0.55714286 0.57142857 0.58571429 0.6 0.61428571 0.62857143 0.64285714 0.65714286 0.67142857 0.68571429 0.7 0.71428571 0.72857143 0.74285714 0.75714286 0.77142857 0.78571429 0.8 0.81428571 0.82857143 0.84285714 0.85714286 0.87142857 0.88571429 0.9 0.91428571 0.92857143 0.94285714 0.95714286 0.97142857 0.98571429 1 1 1 1 1 1
  arc A10 (-17.7816, -18.2774) -> (-16.3186, -19.5947) centre (0, 0) ccw
  spline S5 degree 5 poles (-16.3186, -19.5947) (-16.3046, -19.5907) (-16.2767, -19.5825) (-16.2349, -19.5702) (-16.1792, -19.5535) (-16.1099, -19.5324) (-16.0408, -19.5109) (-15.9719, -19.4891) (-15.9033, -19.467) (-15.8348, -19.4445) (-15.7666, -19.4217) (-15.6986, -19.3986) (-15.6309, -19.3752) (-15.5634, -19.3514) (-15.4961, -19.3273) (-15.4291, -19.3029) (-15.3623, -19.2781) (-15.2957, -19.253) (-15.2295, -19.2276) (-15.1634, -19.2018) (-15.0976, -19.1757) (-15.0321, -19.1492) (-14.9669, -19.1224) (-14.9019, -19.0953) (-14.8372, -19.0678) (-14.7727, -19.04) (-14.7085, -19.0119) (-14.6447, -18.9834) (-14.5811, -18.9545) (-14.5177, -18.9253) (-14.4547, -18.8958) (-14.392, -18.8659) (-14.3296, -18.8356) (-14.2674, -18.805) (-14.2056, -18.7741) (-14.1441, -18.7428) (-14.083, -18.7111) (-14.0221, -18.6791) (-13.9616, -18.6467) (-13.9014, -18.6139) (-13.8415, -18.5808) (-13.782, -18.5473) (-13.7229, -18.5134) (-13.6641, -18.4792) (-13.6057, -18.4445) (-13.5476, -18.4095) (-13.4899, -18.3741) (-13.4326, -18.3383) (-13.3757, -18.3021) (-13.3192, -18.2656) (-13.2631, -18.2286) (-13.2074, -18.1912) (-13.1522, -18.1533) (-13.0975, -18.115) (-13.0433, -18.0763) (-12.9895, -18.0371) (-12.9361, -17.9975) (-12.8831, -17.9576) (-12.8306, -17.9172) (-12.7786, -17.8764) (-12.7272, -17.8351) (-12.6765, -17.7931) (-12.6266, -17.7504) (-12.5775, -17.7071) (-12.5291, -17.6632) (-12.4813, -17.6188) (-12.4338, -17.5742) (-12.3867, -17.5292) (-12.3402, -17.4838) (-12.2947, -17.4376) (-12.2508, -17.39) (-12.2176, -17.3505) (-12.1939, -17.3199) (-12.1787, -17.299) (-12.1713, -17.2884) knots -1 -1 -1 -1 -1 -1 -0.98571429 -0.97142857 -0.95714286 -0.94285714 -0.92857143 -0.91428571 -0.9 -0.88571429 -0.87142857 -0.85714286 -0.84285714 -0.82857143 -0.81428571 -0.8 -0.78571429 -0.77142857 -0.75714286 -0.74285714 -0.72857143 -0.71428571 -0.7 -0.68571429 -0.67142857 -0.65714286 -0.64285714 -0.62857143 -0.61428571 -0.6 -0.58571429 -0.57142857 -0.55714286 -0.54285714 -0.52857143 -0.51428571 -0.5 -0.48571429 -0.47142857 -0.45714286 -0.44285714 -0.42857143 -0.41428571 -0.4 -0.38571429 -0.37142857 -0.35714286 -0.34285714 -0.32857143 -0.31428571 -0.3 -0.28571429 -0.27142857 -0.25714286 -0.24285714 -0.22857143 -0.21428571 -0.2 -0.18571429 -0.17142857 -0.15714286 -0.14285714 -0.12857143 -0.11428571 -0.1 -0.08571429 -0.07142857 -0.05714286 -0.04285714 -0.02857143 -0.01428571 0 0 0 0 0 0
  line L5 (-12.1713, -17.2884) -> (-11.6816, -16.5936)
  arc A11 (-9.6848, -16.1709) -> (-11.6816, -16.5936) centre (-10.4555, -17.4577) ccw
  arc A12 (-9.6848, -16.1709) -> (-9.162, -16.4727) centre (0, 0) ccw
  arc A13 (-8.5297, -18.4134) -> (-9.162, -16.4727) centre (-9.8911, -17.7836) ccw
  line L6 (-8.5297, -18.4134) -> (-8.8866, -19.1849)
  spline S6 degree 5 poles (-8.8866, -19.1849) (-8.892, -19.1966) (-8.9025, -19.2202) (-8.9172, -19.256) (-8.9348, -19.3045) (-8.954, -19.3663) (-8.9713, -19.4288) (-8.9874, -19.4918) (-9.0028, -19.555) (-9.0177, -19.6185) (-9.0322, -19.6821) (-9.046, -19.746) (-9.059, -19.8102) (-9.071, -19.8747) (-9.082, -19.9396) (-9.0922, -20.0048) (-9.1015, -20.0702) (-9.1102, -20.1359) (-9.1183, -20.2017) (-9.1258, -20.2678) (-9.1329, -20.3339) (-9.1393, -20.4003) (-9.1451, -20.4668) (-9.1503, -20.5335) (-9.1549, -20.6005) (-9.1588, -20.6675) (-9.1622, -20.7348) (-9.1651, -20.8022) (-9.1674, -20.8697) (-9.1693, -20.9373) (-9.1706, -21.0051) (-9.1714, -21.073) (-9.1717, -21.1411) (-9.1714, -21.2092) (-9.1707, -21.2775) (-9.1694, -21.3459) (-9.1677, -21.4144) (-9.1655, -21.483) (-9.1628, -21.5518) (-9.1596, -21.6206) (-9.156, -21.6895) (-9.1519, -21.7585) (-9.1474, -21.8276) (-9.1423, -21.8968) (-9.1369, -21.966) (-9.1309, -22.0354) (-9.1246, -22.1048) (-9.1177, -22.1743) (-9.1105, -22.2439) (-9.1028, -22.3135) (-9.0946, -22.3833) (-9.0861, -22.453) (-9.0771, -22.5229) (-9.0676, -22.5928) (-9.0578, -22.6628) (-9.0475, -22.7328) (-9.0368, -22.8029) (-9.0257, -22.873) (-9.0142, -22.9432) (-9.0022, -23.0134) (-8.9899, -23.0837) (-8.9771, -23.154) (-8.964, -23.2243) (-8.9504, -23.2947) (-8.9364, -23.3652) (-8.922, -23.4356) (-8.9073, -23.5061) (-8.8921, -23.5766) (-8.8765, -23.6472) (-8.8606, -23.7178) (-8.8442, -23.7884) (-8.8308, -23.8449) (-8.8206, -23.8873) (-8.8137, -23.9156) (-8.8102, -23.9297) knots 0 0 0 0 0 0 0.01428571 0.02857143 0.04285714 0.05714286 0.07142857 0.08571429 0.1 0.11428571 0.12857143 0.14285714 0.15714286 0.17142857 0.18571429 0.2 0.21428571 0.22857143 0.24285714 0.25714286 0.27142857 0.28571429 0.3 0.31428571 0.32857143 0.34285714 0.35714286 0.37142857 0.38571429 0.4 0.41428571 0.42857143 0.44285714 0.45714286 0.47142857 0.48571429 0.5 0.51428571 0.52857143 0.54285714 0.55714286 0.57142857 0.58571429 0.6 0.61428571 0.62857143 0.64285714 0.65714286 0.67142857 0.68571429 0.7 0.71428571 0.72857143 0.74285714 0.75714286 0.77142857 0.78571429 0.8 0.81428571 0.82857143 0.84285714 0.85714286 0.87142857 0.88571429 0.9 0.91428571 0.92857143 0.94285714 0.95714286 0.97142857 0.98571429 1 1 1 1 1 1
  arc A14 (-8.8102, -23.9297) -> (-6.9379, -24.538) centre (0, 0) ccw
  spline S7 degree 5 poles (-6.9379, -24.538) (-6.9268, -24.5286) (-6.9046, -24.5098) (-6.8714, -24.4815) (-6.8274, -24.4437) (-6.7726, -24.3962) (-6.7182, -24.3485) (-6.6642, -24.3005) (-6.6104, -24.2524) (-6.557, -24.2041) (-6.504, -24.1555) (-6.4513, -24.1067) (-6.3989, -24.0578) (-6.3469, -24.0086) (-6.2953, -23.9592) (-6.244, -23.9096) (-6.193, -23.8598) (-6.1425, -23.8098) (-6.0922, -23.7596) (-6.0424, -23.7092) (-5.9929, -23.6586) (-5.9438, -23.6078) (-5.8951, -23.5568) (-5.8468, -23.5056) (-5.7988, -23.4541) (-5.7513, -23.4025) (-5.7041, -23.3507) (-5.6573, -23.2987) (-5.611, -23.2465) (-5.565, -23.194) (-5.5194, -23.1414) (-5.4743, -23.0886) (-5.4296, -23.0356) (-5.3853, -22.9824) (-5.3414, -22.9289) (-5.2979, -22.8753) (-5.2549, -22.8215) (-5.2124, -22.7675) (-5.1702, -22.7133) (-5.1286, -22.6589) (-5.0874, -22.6043) (-5.0466, -22.5494) (-5.0064, -22.4944) (-4.9666, -22.4392) (-4.9273, -22.3838) (-4.8886, -22.3282) (-4.8503, -22.2724) (-4.8125, -22.2164) (-4.7752, -22.1602) (-4.7384, -22.1038) (-4.7022, -22.0472) (-4.6666, -21.9904) (-4.6316, -21.9334) (-4.5971, -21.8761) (-4.5633, -21.8187) (-4.5301, -21.761) (-4.4974, -21.7031) (-4.4653, -21.6451) (-4.4337, -21.5869) (-4.4028, -21.5285) (-4.3727, -21.4698) (-4.3435, -21.4108) (-4.3153, -21.3515) (-4.288, -21.292) (-4.2617, -21.2322) (-4.236, -21.1722) (-4.2108, -21.1121) (-4.186, -21.0518) (-4.162, -20.9914) (-4.1392, -20.9307) (-4.1185, -20.8694) (-4.1042, -20.8198) (-4.0951, -20.7822) (-4.0897, -20.757) (-4.0872, -20.7443) knots -1 -1 -1 -1 -1 -1 -0.98571429 -0.97142857 -0.95714286 -0.94285714 -0.92857143 -0.91428571 -0.9 -0.88571429 -0.87142857 -0.85714286 -0.84285714 -0.82857143 -0.81428571 -0.8 -0.78571429 -0.77142857 -0.75714286 -0.74285714 -0.72857143 -0.71428571 -0.7 -0.68571429 -0.67142857 -0.65714286 -0.64285714 -0.62857143 -0.61428571 -0.6 -0.58571429 -0.57142857 -0.55714286 -0.54285714 -0.52857143 -0.51428571 -0.5 -0.48571429 -0.47142857 -0.45714286 -0.44285714 -0.42857143 -0.41428571 -0.4 -0.38571429 -0.37142857 -0.35714286 -0.34285714 -0.32857143 -0.31428571 -0.3 -0.28571429 -0.27142857 -0.25714286 -0.24285714 -0.22857143 -0.21428571 -0.2 -0.18571429 -0.17142857 -0.15714286 -0.14285714 -0.12857143 -0.11428571 -0.1 -0.08571429 -0.07142857 -0.05714286 -0.04285714 -0.02857143 -0.01428571 0 0 0 0 0 0
  line L7 (-4.0872, -20.7443) -> (-3.9224, -19.9103)
  arc A15 (-2.2702, -18.712) -> (-3.9224, -19.9103) centre (-2.4509, -20.2011) ccw
  arc A16 (-2.2702, -18.712) -> (-1.6698, -18.7751) centre (0, 0) ccw
  arc A17 (-0.3029, -20.2908) -> (-1.6698, -18.7751) centre (-1.8027, -20.2692) ccw
  line L8 (-0.3029, -20.2908) -> (-0.3151, -21.1407)
  spline S8 degree 5 poles (-0.3151, -21.1407) (-0.3153, -21.1537) (-0.3153, -21.1795) (-0.3142, -21.2182) (-0.3105, -21.2697) (-0.3029, -21.3339) (-0.2933, -21.398) (-0.2824, -21.4621) (-0.2707, -21.5262) (-0.2585, -21.5902) (-0.2459, -21.6543) (-0.2325, -21.7182) (-0.2183, -21.7822) (-0.203, -21.846) (-0.1867, -21.9097) (-0.1694, -21.9734) (-0.1513, -22.037) (-0.1325, -22.1005) (-0.1132, -22.1639) (-0.0932, -22.2273) (-0.0727, -22.2906) (-0.0516, -22.3539) (-0.0299, -22.417) (-0.0075, -22.4801) (0.0156, -22.5431) (0.0392, -22.606) (0.0635, -22.6688) (0.0883, -22.7315) (0.1136, -22.7941) (0.1394, -22.8567) (0.1658, -22.9191) (0.1927, -22.9815) (0.2201, -23.0438) (0.2481, -23.1059) (0.2765, -23.168) (0.3055, -23.23) (0.3349, -23.2919) (0.3648, -23.3537) (0.3952, -23.4154) (0.4261, -23.4769) (0.4575, -23.5384) (0.4893, -23.5998) (0.5215, -23.6611) (0.5543, -23.7222) (0.5874, -23.7833) (0.6211, -23.8442) (0.6551, -23.905) (0.6896, -23.9658) (0.7246, -24.0264) (0.7599, -24.0869) (0.7957, -24.1473) (0.8319, -24.2075) (0.8686, -24.2677) (0.9056, -24.3277) (0.9431, -24.3876) (0.9809, -24.4474) (1.0192, -24.5071) (1.0579, -24.5666) (1.097, -24.626) (1.1364, -24.6853) (1.1763, -24.7445) (1.2166, -24.8035) (1.2572, -24.8625) (1.2982, -24.9212) (1.3396, -24.9799) (1.3814, -25.0384) (1.4236, -25.0968) (1.4662, -25.1551) (1.5091, -25.2132) (1.5524, -25.2712) (1.596, -25.329) (1.6312, -25.3752) (1.6578, -25.4098) (1.6756, -25.4328) (1.6845, -25.4443) knots 0 0 0 0 0 0 0.01428571 0.02857143 0.04285714 0.05714286 0.07142857 0.08571429 0.1 0.11428571 0.12857143 0.14285714 0.15714286 0.17142857 0.18571429 0.2 0.21428571 0.22857143 0.24285714 0.25714286 0.27142857 0.28571429 0.3 0.31428571 0.32857143 0.34285714 0.35714286 0.37142857 0.38571429 0.4 0.41428571 0.42857143 0.44285714 0.45714286 0.47142857 0.48571429 0.5 0.51428571 0.52857143 0.54285714 0.55714286 0.57142857 0.58571429 0.6 0.61428571 0.62857143 0.64285714 0.65714286 0.67142857 0.68571429 0.7 0.71428571 0.72857143 0.74285714 0.75714286 0.77142857 0.78571429 0.8 0.81428571 0.82857143 0.84285714 0.85714286 0.87142857 0.88571429 0.9 0.91428571 0.92857143 0.94285714 0.95714286 0.97142857 0.98571429 1 1 1 1 1 1
  arc A18 (1.6845, -25.4443) -> (3.6424, -25.2385) centre (0, 0) ccw
  spline S9 degree 5 poles (3.6424, -25.2385) (3.6488, -25.2254) (3.6614, -25.1992) (3.6802, -25.1599) (3.7051, -25.1074) (3.7357, -25.0417) (3.766, -24.976) (3.7959, -24.9102) (3.8254, -24.8444) (3.8545, -24.7785) (3.8832, -24.7126) (3.9116, -24.6466) (3.9395, -24.5805) (3.967, -24.5145) (3.9941, -24.4483) (4.0208, -24.3822) (4.047, -24.316) (4.0729, -24.2497) (4.0984, -24.1834) (4.1234, -24.1171) (4.148, -24.0508) (4.1722, -23.9844) (4.1959, -23.9179) (4.2193, -23.8515) (4.2422, -23.785) (4.2646, -23.7185) (4.2866, -23.652) (4.3082, -23.5854) (4.3293, -23.5189) (4.35, -23.4523) (4.3702, -23.3857) (4.39, -23.3191) (4.4093, -23.2524) (4.4281, -23.1858) (4.4464, -23.1192) (4.4643, -23.0525) (4.4817, -22.9858) (4.4986, -22.9192) (4.5151, -22.8525) (4.531, -22.7859) (4.5464, -22.7192) (4.5614, -22.6526) (4.5758, -22.586) (4.5896, -22.5194) (4.603, -22.4528) (4.6158, -22.3862) (4.6281, -22.3196) (4.6398, -22.2531) (4.651, -22.1866) (4.6617, -22.1201) (4.6717, -22.0537) (4.6812, -21.9873) (4.69, -21.9209) (4.6981, -21.8547) (4.7056, -21.7884) (4.7125, -21.7222) (4.7188, -21.6561) (4.7246, -21.59) (4.7298, -21.524) (4.7342, -21.458) (4.7379, -21.3921) (4.7406, -21.3264) (4.7423, -21.2608) (4.7429, -21.1953) (4.7427, -21.1299) (4.7418, -21.0647) (4.7403, -20.9995) (4.7384, -20.9344) (4.7358, -20.8695) (4.7319, -20.8047) (4.7259, -20.7403) (4.7188, -20.6892) (4.7119, -20.6511) (4.7065, -20.6258) (4.7036, -20.6132) knots -1 -1 -1 -1 -1 -1 -0.98571429 -0.97142857 -0.95714286 -0.94285714 -0.92857143 -0.91428571 -0.9 -0.88571429 -0.87142857 -0.85714286 -0.84285714 -0.82857143 -0.81428571 -0.8 -0.78571429 -0.77142857 -0.75714286 -0.74285714 -0.72857143 -0.71428571 -0.7 -0.68571429 -0.67142857 -0.65714286 -0.64285714 -0.62857143 -0.61428571 -0.6 -0.58571429 -0.57142857 -0.55714286 -0.54285714 -0.52857143 -0.51428571 -0.5 -0.48571429 -0.47142857 -0.45714286 -0.44285714 -0.42857143 -0.41428571 -0.4 -0.38571429 -0.37142857 -0.35714286 -0.34285714 -0.32857143 -0.31428571 -0.3 -0.28571429 -0.27142857 -0.25714286 -0.24285714 -0.22857143 -0.21428571 -0.2 -0.18571429 -0.17142857 -0.15714286 -0.14285714 -0.12857143 -0.11428571 -0.1 -0.08571429 -0.07142857 -0.05714286 -0.04285714 -0.02857143 -0.01428571 0 0 0 0 0 0
  line L9 (4.7036, -20.6132) -> (4.515, -19.7844)
  arc A19 (5.5369, -18.0176) -> (4.515, -19.7844) centre (5.9775, -19.4515) ccw
  arc A20 (5.5369, -18.0176) -> (6.111, -17.8311) centre (0, 0) ccw
  arc A21 (7.9763, -18.6597) -> (6.111, -17.8311) centre (6.5974, -19.2501) ccw
  line L10 (7.9763, -18.6597) -> (8.3108, -19.4412)